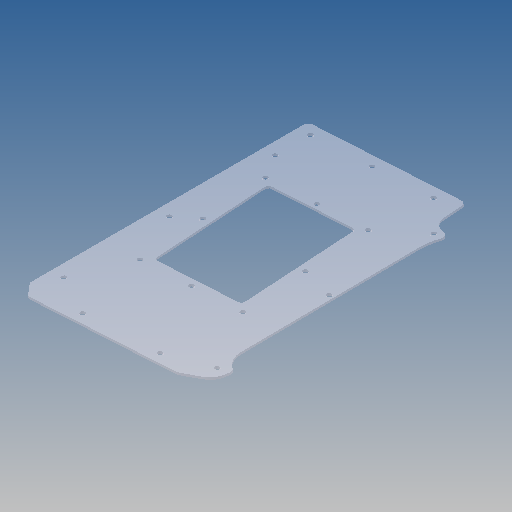
# Autodesk Inventor part: J009837
Saved by Autodesk Inventor 2020.3 (Build 243373000, 373)
## iProperties
RuleStatus: InUse
AfterDocSave0: file://Part Number Cleaner
Created: 2019-09-16
Material: POLYCARBONATE, CLEAR
Vendor: HHMI: JRC - ID&F
Document SubType Name: Sheet Metal
Designer: goulett
Density: 1.2 g/cm^3
Appearance: Polycarbonate (Clear)
Sheet Metal Rule: Default
Description: SLANTED FACE OF THE RAT CAGE LID WITH A CUT OUT FOR THE BOTTLE HOLDER
Project: P-342901
Part Number: J009837
LAB/DEPT: VIVARIUM (SHARED RESOURCES)
REQUESTING SCIENTIST: COX, JAMES
SURFACE ROUGHNESS: N/A
DESIGN DEPARTMENT: HHMI: JRC - ID&F
SPECIAL FINISH: N/A
ALTERED ITEM PART NUMBER: N/A
ALTERED ITEM VENDOR: N/A
ALTERED ITEM DESCRIPTION: N/A
Author: goulett
Revision Number: -
Autodesk Inventor part; units mm, degrees
ref_plane "YZ Plane" through (0, 0, 0) normal (1, 0, 0) x (0, 1, 0)
ref_plane "XZ Plane" through (0, 0, 0) normal (0, 1, 0) x (-1, 0, 0)
ref_plane "XY Plane" through (0, 0, 0) normal (0, 0, 1) x (1, 0, 0)
sketch "Sketch1" plane through (0, 0, 0) normal (0, 1, 0) x (-1, 0, 0)
  line L0 (-107.4651, -6.5728) -> (-108.712, 11.2585)
  arc A0 (-108.712, 11.2585) -> (-117.5803, 19.5283) centre (-117.5803, 10.6383) ccw
  line L1 (-117.5803, 19.5283) -> (-120.65, 19.5283)
  line L2 (-120.65, 19.5283) -> (-120.65, 24.13)
  arc A1 (-120.65, 24.13) -> (-118.2535, 38.6966) centre (-161.4319, 38.3198) ccw
  line L3 (-128.333, 181.8469) -> (-127, 193.5462)
  line L4 (-109.22, 203.2) -> (-7.62, 209.4141)
  arc A2 (-119.38, 167.7774) -> (-128.333, 181.8469) centre (-135.1274, 167.64) ccw
  line L5 (-107.4651, -6.5728) -> (0, 0)
  line L6 (-7.62, 209.4141) -> (0, 200.333)
  line L7 (0, 0) -> (0, 200.333)
  line L8 (-109.22, 203.2) -> (-127, 193.5462)
  line L9 (-118.2535, 38.6966) -> (-119.38, 167.7774)
  line L10 (0, 0) -> (-88.3844, 0) construction
  line L11 (-8.89, 7.0905) -> (-8.89, 184.8905) construction
  line L12 (-8.89, 7.0905) -> (-92.5537, 1.9734) construction
  line L13 (-114.808, 24.1003) -> (-115.616, 100.296) construction
  line L14 (-114.808, 24.1003) -> (-120.65, 186.0215) construction
  line L15 (32.2864, 0) -> (-193.7183, 0) construction
  line L16 (-38.1, 200.4246) -> (-90.8335, 197.1993) construction
  line L17 (-58.42, 206.3071) -> (-51.3909, 91.3828) construction
  point P0 (-50.7218, 4.532)
  point P1 (-8.89, 108.6905)
  point P2 (-8.89, 32.4905)
  dimension "d52" = 76.2
  dimension "d54" = 76.2
  dimension "d98" = 25
  dimension "d99" = 55
  dimension "d100" = 86.5
  dimension "d103" = 8.89
  dimension "d104" = 7.62
  dimension "d106" = 203.2
  dimension "d108" = 127
  dimension "d109" = 109.22
  dimension "d111" = 167.64
  dimension "d112" = 120.65
  dimension "d114" = 41.91
  dimension "d115" = 41.91
  dimension "d117" = 3.175
  dimension "d118" = 76.2
  dimension "d121" = 4.572
  dimension "d122" = 8.89
  dimension "d123" = 86
  dimension "d124" = 43.18
  dimension "d125" = 15.748
  dimension "d127" = 52.832
  dimension "d128" = 7.112
  dimension "d129" = 38.1
  dimension "d130" = 140
  dimension "d131" = 7.62
  dimension "d159" = 25.4
  dimension "d160" = 119.38
  dimension "d163" = 24.13
  dimension "d166" = 3
  dimension "d169" = 120.65
  dimension "d170" = 108.712
  dimension "d172" = 26.67
  dimension "d174" = 193.04
  dimension "d175" = 114.808
  constraints: 34 end point, 8 point on circle, 4 parallel, 4 tangent, 3 centre point, 3 point on line, 2 midpoint, 2 perpendicular, 2 vertical, 1 coincident, 1 horizontal
  measures "d52" distance of point (-8.89, 108.691) L11.end
  measures "d54" distance of point (-8.89, 32.491) point (-8.89, 108.691)
  measures "d98" angle of L8 L4
  measures "d99" angle of L8 L3
  measures "d100" angle of L7 L4
  measures "d103" distance between parallel lines of L7 L11
  measures "d104" distance between parallel lines of L5 L12
  measures "d106" distance from line of L15 L4.start
  measures "d108" distance from line of L3.end L7
  measures "d109" distance from line of L7 L4.start
  measures "d111" distance from line of A2.centre L15
  measures "d112" distance from line of L7 L14.end
  measures "d114" distance of point (-50.722, 4.532) L11.start
  measures "d115" distance of L12.end point (-50.722, 4.532)
  measures "d117" distance from line of L9 L13.end
  measures "d118" distance of L13.start L13.end
  measures "d121" distance from line of L1 L13.start
  measures "d122" radius of A0
  measures "d123" angle of L0 L15
  measures "d124" radius of A1
  measures "d125" radius of A2
  measures "d127" distance of L16.start L16.end
  measures "d128" distance between parallel lines of L4 L16
  measures "d129" distance from line of L16.start L7
  measures "d130" angle of L7 L6
  measures "d131" distance from line of L7 L4.end
  measures "d159" distance of point (-8.89, 32.491) L11.start
  measures "d160" distance from line of L7 L9.end
  measures "d163" distance from line of L2.end L15
  measures "d166" angle of L17 L9
  measures "d169" distance between parallel lines of L7 L2
  measures "d170" distance from line of L7 L0.end
  measures "d172" distance from line of L5 L1.start
  measures "d174" distance from line of L5 L14.end
  measures "d175" distance from line of L7 L13.start
extrude "Plate1" add sketch "Sketch1" along normal blind 1.5875
fillet "Corner Round1" radius 3.175 7 edges at (0, 0.7937, 200.333) (7.62, 0.7937, 209.4141) (120.65, 0.7937, 24.13) (120.65, 0.7937, 19.5283) (107.4651, 0.7937, -6.5728) (128.333, 0.7937, 181.8469) (0, 0.7937, 0)
fillet "Corner Round1" radius 10.16 1 edges at (109.22, 0.7937, 203.2)
fillet "Corner Round1" radius 12.7 1 edges at (127, 0.7937, 193.5462)
hole "Hole1" at (8.89, 0, 184.8905) at (38.1, 0, 200.4246) at (90.8335, 0, 197.1993) at (120.65, 0, 186.0215) at (115.616, 0, 100.296) at (114.808, 0, 24.1003) at (50.7218, 0, 4.532) at (92.5537, 0, 1.9734) at (8.89, 0, 7.0905) at (8.89, 0, 108.6905) at (8.89, 0, 32.4905) direction (0, 1, 0) diameter 3.4544 end through all
sketch "Sketch4" plane through (0, 1.5875, 0) normal (0, 1, 0) x (1, 0, 0)
  line L0 (24.6883, -53.4312) -> (84.2666, -49.782)
  line L1 (84.2666, -49.782) -> (89.624, -137.2481)
  line L2 (89.624, -137.2481) -> (30.0456, -140.8973)
  line L3 (30.0456, -140.8973) -> (24.6883, -53.4312)
  line L4 (19.3849, -49.9389) -> (89.1042, -45.6686) construction
  line L5 (89.1042, -45.6686) -> (95.005, -142.008) construction
  line L6 (95.005, -142.008) -> (25.2857, -146.2783) construction
  line L7 (25.2857, -146.2783) -> (19.3849, -49.9389) construction
  line L8 (26.1112, -55.8888) -> (83.1543, -52.3949) construction
  line L9 (83.1543, -52.3949) -> (88.2787, -136.0581) construction
  line L10 (88.2787, -136.0581) -> (31.2356, -139.552) construction
  line L11 (31.2356, -139.552) -> (26.1112, -55.8888) construction
  line L12 (0, -199.1774) -> (0, -2.9867) construction
  line L13 (2.9812, 0.1823) -> (104.3236, 6.3807) construction
  point P0 (0, 0)
  point P1 (60.1454, -144.1432)
  point P2 (54.2445, -47.8037)
  point P3 (92.0546, -93.8383)
  point P4 (22.3353, -98.1086)
  dimension "d134" = 6.35
  dimension "d135" = 6.35
  dimension "d136" = 6.35
  dimension "d137" = 6.35
  dimension "d138" = 2.54
  dimension "d139" = 1.27
  dimension "d140" = 1.27
  dimension "d141" = 1.27
  dimension "d142" = 83.82
  dimension "d143" = 57.15
  dimension "d144" = 26.1112
  dimension "d145" = 57.3786
  dimension "d146" = 3.505
  dimension "d149" = 96.52
  constraints: 24 end point, 8 parallel, 4 coincident, 4 midpoint, 3 perpendicular
  measures "d134" distance between parallel lines of L8 L4
  measures "d135" distance between parallel lines of L5 L9
  measures "d136" distance between parallel lines of L7 L11
  measures "d137" distance between parallel lines of L6 L10
  measures "d138" distance between parallel lines of L8 L0
  measures "d139" distance between parallel lines of L1 L9
  measures "d140" distance between parallel lines of L3 L11
  measures "d141" distance between parallel lines of L2 L10
  measures "d142" distance between parallel lines of L10 L8
  measures "d143" distance between parallel lines of L9 L11
  measures "d144" distance from line of L12 L8.start
  measures "d145" distance from line of L8.start L13
  measures "d146" angle of L11 L12
  measures "d149" distance between parallel lines of L4 L6
extrude "Cut2" cut sketch "Sketch4" against normal blind 1.5875
hole "Hole3" at (19.3849, 1.5875, 49.9389) at (89.1042, 1.5875, 45.6686) at (95.005, 1.5875, 142.008) at (25.2857, 1.5875, 146.2783) at (60.1454, 1.5875, 144.1432) at (54.2445, 1.5875, 47.8037) at (92.0546, 1.5875, 93.8383) at (22.3353, 1.5875, 98.1086) direction (0, -1, 0) diameter 3.4544 end through all
fillet "Corner Round3" radius 2.54 4 edges at (84.2666, 0.7937, 49.782) (24.6883, 0.7937, 53.4312) (30.0456, 0.7937, 140.8973) (89.624, 0.7937, 137.2481)
equation "\"d60\" = Thickness"
equation "\"d49\" = Thickness"
equation "\"BendReliefWidth\" = Thickness"
equation "\"BendReliefDepth\" = 0.5 * Thickness"
equation "\"CornerReliefSize\" = 4 * Thickness"
equation "\"MinimumRemnant\" = 2 * Thickness"
equation "\"TransitionRadius\" = BendRadius"
equation "\"JacobiRadiusSize\" = BendRadius"
equation "\"GapSize\" = Thickness"
equation "\"Thickness\" = 1.5875"
equation "\"BendRadius\" = 0.762"
body "Solid1"
